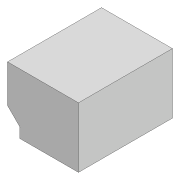
# Autodesk Inventor part: caja area de trabajo
Saved by Autodesk Inventor 2021 (Build 250183000, 183)
## iProperties
Created: 2021-04-14
Part Number: caja area de trabajo
Material: Genérico
Document SubType Name: Modeling
Designer: Admin
Density: 1 g/cm^3
Appearance: Valor por defecto
Author: Admin
Autodesk Inventor part; units mm, degrees
ref_plane "YZ Plane" through (0, 0, 0) normal (1, 0, 0) x (0, 1, 0)
ref_plane "XZ Plane" through (0, 0, 0) normal (0, 1, 0) x (-1, 0, 0)
ref_plane "XY Plane" through (0, 0, 0) normal (0, 0, 1) x (1, 0, 0)
sketch "Boceto1" plane through (0, 0, 0) normal (0, 0, 1) x (1, 0, 0)
  line L0 (0, 340) -> (400, 340)
  line L1 (400, 340) -> (400, 0)
  line L2 (70, 0) -> (70, 56.12)
  line L3 (0, 340) -> (0, 126)
  line L4 (0, 126) -> (70, 56.12)
  line L5 (0, 126) -> (0, 340)
  line L6 (70, 0) -> (400, 0)
  point P0 (0, 0)
  dimension "d0" = 340
  dimension "d1" = 400
  dimension "d2" = 70
  dimension "d3" = 56.12
  dimension "d4" = 214
  constraints: 14 end point, 1 horizontal, 1 perpendicular
  measures "d0" distance of point (0, 0) L0.start
  measures "d1" distance of L0.start L0.end
  measures "d2" distance of point (0, 0) L2.start
  measures "d3" distance of L2.start L2.end
  measures "d4" distance of L0.start L3.end
extrude "Extrusión1" add sketch "Boceto1" along normal blind 530
